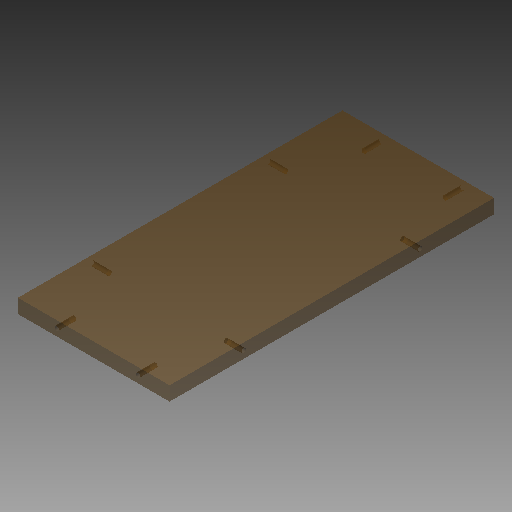
# Autodesk Inventor part: Wand5
Saved by Autodesk Inventor 2018 (Build 220112000, 112)
## iProperties
Created: 2013-02-21
Part Number: Wand5
Material: Polycarbonate, Smoke
Document SubType Name: Modeling
Designer: Neef
Mass: 151.91 g
Surface Area: 359.68 cm^2
Volume: 126.592 cm^3
Density: 1.2 g/cm^3
Appearance: Polycarbonate - Smoked
Author: Neef
Autodesk Inventor part; units mm, degrees
ref_plane "YZ Plane" through (0, 0, 0) normal (1, 0, 0) x (0, 1, 0)
ref_plane "XZ Plane" through (0, 0, 0) normal (0, 1, 0) x (-1, 0, 0)
ref_plane "XY Plane" through (0, 0, 0) normal (0, 0, 1) x (1, 0, 0)
sketch "Skizze1" plane through (0, 0, 0) normal (0, 0, 1) x (1, 0, 0)
  line L0 (0, 128.8) -> (0, -128.8) projected
  line L1 (-60.2, 0) -> (60.2, 0) projected
  line L2 (43, 92) -> (-43, 92)
  line L3 (-43, 92) -> (-43, -92)
  line L4 (-43, -92) -> (43, -92)
  line L5 (43, -92) -> (43, 92)
  point P0 (0, 0)
  point P1 (43, 0)
  point P2 (0, 92)
  dimension "d0" = 184
  dimension "d1" = 86
  constraints: 8 end point, 2 midpoint, 2 parallel, 2 point on line, 1 horizontal, 1 perpendicular
  measures "d0" distance of L4.end L2.start
  measures "d1" distance of L2.start L2.end
extrude "Extrusion1" add sketch "Skizze1" along normal blind 8
sketch "Skizze2" plane through (-43, -92, 0) normal (-1, 0, 0) x (0, 0, 1)
  circle A0 centre (-277.5, 142) radius 3.1 projected
  circle A1 centre (-52, 188) radius 3.1 projected
  circle A2 centre (-221.5, 188) radius 3.1 projected
  circle A3 centre (4, 142) radius 3.1 projected
  circle A4 centre (-277.5, 42) radius 3.1 projected
  circle A5 centre (4, 42) radius 3.1 projected
  circle A6 centre (-221.5, -4) radius 3.1 projected
  circle A7 centre (-52, -4) radius 3.1 projected
  line L0 (8, 192) -> (8, -8) projected
  line L1 (8, 192) -> (-281.5, 192) projected
  line L2 (-281.5, 192) -> (-281.5, 115) projected
  line L3 (-281.5, 115) -> (-333.5, 115) projected
  line L4 (-333.5, 115) -> (-333.5, 69) projected
  line L5 (-281.5, 69) -> (-333.5, 69) projected
  line L6 (-281.5, -8) -> (-281.5, 69) projected
  line L7 (8, -8) -> (-281.5, -8) projected
  point P0 (0, 92)
  constraints: 2 coincident
hole "Bohrung1" at (-43, 50, 4) at (-43, -50, 4) direction (1, 0, 0) diameter 2.459 depth 10 tip angle 118 thread size "M3x0.5" class "6H" standard "ISO Metric profile"
sketch "Skizze3" plane through (-43, 92, 0) normal (0, 1, 0) x (1, 0, 0)
  circle A0 centre (68, -4) radius 3.1 projected
  circle A1 centre (22, -4) radius 3.1 projected
  line L0 (0, -8) -> (0, 273.5) projected
  line L1 (86, -8) -> (0, -8) projected
  line L2 (86, 273.5) -> (86, -8) projected
  line L3 (0, 273.5) -> (86, 273.5) projected
  point P0 (43, 0)
  constraints: 2 coincident
hole "Bohrung2" at (-21, 92, 4) at (25, 92, 4) direction (0, -1, 0) diameter 2.459 depth 10 tip angle 118 thread size "M3x0.5" class "6H" standard "ISO Metric profile"
mirror "Spiegeln1" about plane through (0, 0, 0) normal (0, 1, 0) of "Bohrung2"
sketch "Skizze4" plane through (43, -92, 0) normal (1, 0, 0) x (0, 0, -1)
  circle A0 centre (-4, 142) radius 3.1 projected
  circle A1 centre (-4, 42) radius 3.1 projected
  point P0 (0, 92)
  constraints: 2 coincident
hole "Bohrung3" at (43, 50, 4) at (43, -50, 4) direction (-1, 0, 0) diameter 2.459 depth 10 tip angle 118 thread size "M3x0.5" class "6H" standard "ISO Metric profile"
